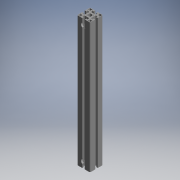
# Autodesk Inventor part: HFS8-5050-500-LSV-RSV
Saved by Autodesk Inventor 2017.3 (Build 213256000, 256)
## iProperties
Part Number: HFS8-5050-500-LSV-RSV
Material: Generic
Catalog Web Link: www.cadenas.de
Description: NEFS8-5050, EFS8-5050, EFSB8-5050, HFS8-5050, HFSB8-5050, GFS8-5050, HFSF8-5050, HFST8-5050-HFS8 Series Aluminum Extrusions 50 Square -1 Slot-
Vendor: MISUMI
Document SubType Name: Modeling
Designer: partserver
Manufacturer: MISUMI
Mass: 622.053 g
Surface Area: 2899.68 cm^2
Volume: 622.053 cm^3
Density: 1 g/cm^3
Appearance: PSOLRGB-175-175-175
Category: PARTsolutions
Company: MISUMI
Title: HFS8-5050-500-LSV-RSV
Author: Cadenas PARTsolutions
Comments: HFS8 Series Aluminum Extrusions 50 Square -1 Slot-
PSOL_IDENT_0: {$CADENAS_DATA\23d-libs\misumi\metric\38_al_extrusions_blackets\8_45\hfs8_5050.prj},643 {VTYP=3D},{N
PSOL_IDENT_1: B=HFS8-5050-500-LSV-RSV},{LINA=HFS8-5050-500-LSV-RSV},{NN=NEFS8-5050, EFS8-5050, EFSB8-5050, HFS8-50
PSOL_IDENT_2: 50, HFSB8-5050, GFS8-5050, HFSF8-5050, HFST8-5050},{DATE=08.06.2021 08:26:18},{GEOMDATE=13.07.2020 0
PSOL_IDENT_3: 4:45:18},{VERSION=},{LINEID=130},{WBVAR=L,ALT1,ALT2,ALT4,ALT5,CP5,DL5,DR5,ALT6,ALT9,ALT10,ALT11,HP6,
PSOL_IDENT_4: NHL6,DL6,NHR6,DR6,ALT7,ALT8,NH9,AH,BH,CH,DH,EH,NH10,AV,BV,CV,DV,EV,NH11,AP,BP,CP,DP,EP,ALT12,ALT13,Z
PSOL_IDENT_5: ,NH12,XA,XB,XC,XD,XE,NH13,YA,YB,YC,YD,YE,ALT14,HP14,DL14,DR14,ALT15,HP15,DL15,DR15,ALT16,HP16,DL16,D
PSOL_IDENT_6: R16,ALT19,ALT20},{WBNUMERIC=L,NH9,AH,BH,CH,DH,EH,NH10,AV,BV,CV,DV,EV,NH11,AP,BP,CP,DP,EP,NH12,XA,XB,
PSOL_IDENT_7: XC,XD,XE,NH13,YA,YB,YC,YD,YE}  {NB=HFS8-5050-500-LSV-RSV},{LINA=HFS8-5050-500-LSV-RSV},{KT=DUMMY},{P
PSOL_IDENT_8: N=HFS8-5050-500-LSV-RSV},{TPS=HFS8-5050},{MAT=A6N01SS-T5 Aluminum Alloy},{ST=Clear Anodize},{FRMW=50
PSOL_IDENT_9: },{FRMH=50},{FRD=12.5},{L=500.0},{MASS=3.43},{SA=1150},{LX=26.64x10^4},{LY=26.64x10^4},{ALT1=},{M1=0
PSOL_IDENT_10: },{IDM1=10.106},{DPL1=0},{DPR1=0},{ALT1PN=},{ALT2=},{ALT2ALG= '','w/o End Tapping (Heli-Coil Insert)'
PSOL_IDENT_11: ,'LHP','with LHP (Tapping on the Left (Heli-Coil Insert))','RHP','with RHP (Tapping on the Right (He
PSOL_IDENT_12: li-Coil Insert))','HPW','with HPW (Tapping on Both Ends (Heli-Coil Insert))' },{M2=0},{DP2=0},{ALT2P
PSOL_IDENT_13: N=},{ALT4=},{ALT4ALG= '', 'w/o SC (High Precision Cut)', 'SC', 'with SC (High Precision Cut)' },{ALT
PSOL_IDENT_14: 4PN=},{ALT5=},{ALT5ALG= '','w/o 45 Degree Cut','1','with 45 Degree Cut' },{CP5=},{CP5ALG= '','N/A' }
PSOL_IDENT_15: ,{DL5=},{DL5ALG= '','N/A' },{DR5=},{DR5ALG= '','N/A' },{FRMLALT5=0},{FRMRALT5=0},{ALT5PN=},{ALT6=},{
PSOL_IDENT_16: ALT6ALG= '','w/o Fastening Location Wrench Access Hole Alterations','1','with Fastening Location Wre
PSOL_IDENT_17: nch Access Hole Alterations' },{ALT9=},{ALT9ALG= '','w/o Location Specified Wrench Access Hole Alter
PSOL_IDENT_18: atons (Horizontal)','1','with Location Specified Wrench Access Hole Alteratons (Horizontal)' },{ALT1
PSOL_IDENT_19: 0=},{ALT10ALG= '','w/o Location Specified Wrench Access Hole Alteratons (Vertical)','1','with Locati
PSOL_IDENT_20: on Specified Wrench Access Hole Alteratons (Vertical)' },{ALT11=},{ALT11ALG= '','w/o Location Specif
PSOL_IDENT_21: ied Wrench Access Hole Alteratons (Crisscross)','1','with Location Specified Wrench Access Hole Alte
PSOL_IDENT_22: ratons (Crisscross)' },{HP6=},{HP6ALG= '','N/A' },{NHL6=},{NHL6ALG= '','N/A' },{DL6=},{DL6ALG= '','N
PSOL_IDENT_23: /A' },{NHR6=},{NHR6ALG= '','N/A' },{DR6=},{DR6ALG= '','N/A' },{HL6=0.0},{HL6D=0.0},{HR6=0.0},{HR6D=0
PSOL_IDENT_24: .0},{J6=0},{J6D=0},{K6=0},{K6D=0},{DD6=0},{DD6ALG=0},{ALT7=},{ALT7ALG= '','N/A' },{ALT8=},{ALT8ALG= ''
PSOL_IDENT_25: ,'N/A' },{ALT678PN=},{NH9=0},{NH9MAX=5},{NH9ALG=[0]},{AH=0.0},{AHMIN=7},{AHMAX=495},{AHALG=[0]},{BH=
PSOL_IDENT_26: 0.0},{BHMIN=2},{BHMAX=497},{BHALG=[0]},{CH=0.0},{CHMIN=2},{CHMAX=499},{CHALG=[0]},{DH=0.0},{DHMIN=2}
PSOL_IDENT_27: ,{DHMAX=501},{DHALG=[0]},{EH=0.0},{EHMIN=2},{EHMAX=493},{EHALG=[0]},{NH10=0},{NH10MAX=5},{NH10ALG=[0
PSOL_IDENT_28: ]},{AV=0.0},{AVMIN=7},{AVMAX=495},{AVALG=[0]},{BV=0.0},{BVMIN=2},{BVMAX=497},{BVALG=[0]},{CV=0.0},{C
PSOL_IDENT_29: VMIN=2},{CVMAX=499},{CVALG=[0]},{DV=0.0},{DVMIN=2},{DVMAX=501},{DVALG=[0]},{EV=0.0},{EVMIN=2},{EVMAX=
PSOL_IDENT_30: 493},{EVALG=[0]},{NH11=0},{NH11MAX=5},{NH11ALG=[0]},{AP=0.0},{APMIN=7},{APMAX=495},{APALG=[0]},{BP=0
PSOL_IDENT_31: .0},{BPMIN=2},{BPMAX=497},{BPALG=[0]},{CP=0.0},{CPMIN=2},{CPMAX=499},{CPALG=[0]},{DP=0.0},{DPMIN=2},
PSOL_IDENT_32: {DPMAX=501},{DPALG=[0]},{EP=0.0},{EPMIN=2},{EPMAX=493},{EPALG=[0]},{ALT9PN=},{ALT10PN=},{ALT11PN=},{
PSOL_IDENT_33: ALT91011PN=},{ALT12=},{ALT12ALG= '','w/o Counterbore Hole in Specified Position (Vertical)','1','wit
PSOL_IDENT_34: h Counterbore Hole in Specified Position (Vertical)' },{ALT13=},{ALT13ALG= '','w/o Counterbore Hole
PSOL_IDENT_35: in Specified Position (Horizontal)','1','with Counterbore Hole in Specified Position (Horizontal)' }
PSOL_IDENT_36: ,{Z=},{ZALG= '','N/A' },{DD12=0.0},{DD112=0},{NH12=0},{NH12MAX=5},{NH12ALG=[0]},{XA=0.0},{XAMIN=7},{
PSOL_IDENT_37: XAMAX=495},{XAALG=[0]},{XB=0.0},{XBMIN=2},{XBMAX=497},{XBALG=[0]},{XC=0.0},{XCMIN=2},{XCMAX=499},{XC
PSOL_IDENT_38: ALG=[0]},{XD=0.0},{XDMIN=2},{XDMAX=501},{XDALG=[0]},{XE=0.0},{XEMIN=2},{XEMAX=493},{XEALG=[0]},{NH13=
PSOL_IDENT_39: 0},{NH13MAX=5},{NH13ALG=[0]},{YA=0.0},{YAMIN=7},{YAMAX=495},{YAALG=[0]},{YB=0.0},{YBMIN=2},{YBMAX=49
PSOL_IDENT_40: 7},{YBALG=[0]},{YC=0.0},{YCMIN=2},{YCMAX=499},{YCALG=[0]},{YD=0.0},{YDMIN=2},{YDMAX=501},{YDALG=[0]}
PSOL_IDENT_41: ,{YE=0.0},{YEMIN=2},{YEMAX=493},{YEALG=[0]},{ALT12PN=},{ALT13PN=},{ALT1213PN=},{ALT14=},{ALT14ALG= ''
PSOL_IDENT_42: ,'w/o D Type Hole Alteration','1','with D Type Hole Alteration' },{HP14=},{HP14ALG= '','N/A' },{DL14=
PSOL_IDENT_43: },{DL14ALG= '','N/A' },{DR14=},{DR14ALG= '','N/A' },{H14=0.0},{D14=0.0},{ALT14PN=},{ALT15=1},{ALT15A
PSOL_IDENT_44: LG= '','w/o S Type Hole Alteration','1','with S Type Hole Alteration' },{HP15=LR},{HP15ALG= 'L','Lef
PSOL_IDENT_45: t','R','Right','LR','Both Sides' },{DL15=V},{DL15ALG= 'H','Horizontal','V','Vertical','P','Crisscros
PSOL_IDENT_46: s' },{DR15=V},{DR15ALG= 'H','Horizontal','V','Vertical','P','Crisscross' },{H15=22.5},{D115=20},{D21
PSOL_IDENT_47: 5=15.1},{ALT15PN=-LSV-RSV},{ALT16=},{ALT16ALG= '','w/o M Type Hole Alteration','1','with M Type Hole
PSOL_IDENT_48: Alteration' },{HP16=},{HP16ALG= '','N/A' },{DL16=},{DL16ALG= '','N/A' },{DR16=},{DR16ALG= '','N/A'
PSOL_IDENT_49: },{H116=0},{D16=0.0},{ALT16PN=},{ALT19=},{ALT19ALG= '','N/A' },{M19=0},{DP19=0},{ALT19PN=},{ALT20=},
PSOL_IDENT_50: {ALT20PN=},{ERRORALT01=OK},{ERRORALT02=OK},{ERRORALT05=OK},{ERRORALT06091=OK},{ERRORALT06092=OK},{ER
PSOL_IDENT_51: RORALT06093=OK},{ERRORALT06094=OK},{ERRORALT06101=OK},{ERRORALT06102=OK},{ERRORALT06103=OK},{ERRORAL
PSOL_IDENT_52: T06104=OK},{ERRORALT06111=OK},{ERRORALT06112=OK},{ERRORALT06113=OK},{ERRORALT06114=OK},{ERRORALT0612
PSOL_IDENT_53: 1=OK},{ERRORALT06122=OK},{ERRORALT06123=OK},{ERRORALT06124=OK},{ERRORALT06131=OK},{ERRORALT06132=OK}
PSOL_IDENT_54: ,{ERRORALT06133=OK},{ERRORALT06134=OK},{ERRORALT0614=OK},{ERRORALT0615=OK},{ERRORALT0616=OK},{ERRORA
PSOL_IDENT_55: LT0619=OK},{ERRORALT0911=OK},{ERRORALT0913=OK},{ERRORALT0914=OK},{ERRORALT0915=OK},{ERRORALT0916=OK}
PSOL_IDENT_56: ,{ERRORALT0919=OK},{ERRORALT1011=OK},{ERRORALT1012=OK},{ERRORALT1014=OK},{ERRORALT1015=OK},{ERRORALT
PSOL_IDENT_57: 1016=OK},{ERRORALT1019=OK},{ERRORALT1112=OK},{ERRORALT1113=OK},{ERRORALT1114=OK},{ERRORALT1115=OK},{
PSOL_IDENT_58: ERRORALT1116=OK},{ERRORALT1119=OK},{ERRORALT1214=OK},{ERRORALT1215=OK},{ERRORALT1216=OK},{ERRORALT12
PSOL_IDENT_59: 19=OK},{ERRORALT1314=OK},{ERRORALT1315=OK},{ERRORALT1316=OK},{ERRORALT1319=OK},{ERRORALT1415=OK},{ER
PSOL_IDENT_60: RORALT1416=OK},{ERRORALT1419=OK},{ERRORALT1516=OK},{ERRORALT1519=OK},{ERRORALT1619=OK},{ERRORPN=},{T
PSOL_IDENT_61: FH=0},{TFW=0}
NB: HFS8-5050-500-LSV-RSV
NN: NEFS8-5050, EFS8-5050, EFSB8-5050, HFS8-5050, HFSB8-5050, GFS8-5050, HFSF8-5050, HFST8-5050
NT: HFS8 Series Aluminum Extrusions 50 Square -1 Slot-
NBSYN: $PN.
LINA: HFS8-5050-500-LSV-RSV
CATALOG: Misumi
PN: HFS8-5050-500-LSV-RSV
TPS: HFS8-5050
MAT: A6N01SS-T5 Aluminum Alloy
ST: Clear Anodize
L: 500
MASS: 3.43
SA: 1150
LX: 26.64x10^4
LY: 26.64x10^4
ALT1: w/o End Tapping
M1: 0
DPL1: 0
DPR1: 0
ALT2: w/o End Tapping (Heli-Coil Insert)
M2: 0
DP2: 0
ALT4: w/o SC (High Precision Cut)
ALT5: w/o 45 Degree Cut
CP5: N/A
DL5: N/A
DR5: N/A
ALT6: w/o Fastening Location Wrench Access Hole Alterations
ALT9: w/o Location Specified Wrench Access Hole Alteratons (Horizontal)
ALT10: w/o Location Specified Wrench Access Hole Alteratons (Vertical)
ALT11: w/o Location Specified Wrench Access Hole Alteratons (Crisscross)
HP6: N/A
NHL6: N/A
DL6: N/A
NHR6: N/A
DR6: N/A
HL6D: 0
HR6D: 0
J6D: 0
K6D: 0
DD6: 0
ALT7: N/A
ALT8: N/A
NH9: 0
AH: 0
BH: 0
CH: 0
DH: 0
EH: 0
NH10: 0
AV: 0
BV: 0
CV: 0
DV: 0
EV: 0
NH11: 0
AP: 0
BP: 0
CP: 0
DP: 0
EP: 0
ALT12: w/o Counterbore Hole in Specified Position (Vertical)
ALT13: w/o Counterbore Hole in Specified Position (Horizontal)
Z: N/A
DD12: 0
DD112: 0
NH12: 0
XA: 0
XB: 0
XC: 0
XD: 0
XE: 0
NH13: 0
YA: 0
YB: 0
YC: 0
YD: 0
YE: 0
ALT14: w/o D Type Hole Alteration
HP14: N/A
DL14: N/A
DR14: N/A
H14: 0
D14: 0
ALT15: with S Type Hole Alteration
HP15: Both Sides
DL15: Vertical
DR15: Vertical
H15: 22.5
D115: 20
D215: 15.1
ALT16: w/o M Type Hole Alteration
HP16: N/A
DL16: N/A
DR16: N/A
H116: 0
D16: 0
ALT19: N/A
M19: 0
DP19: 0
ALT20: w/o CW (End Face C Chamfering)
SUPPLIER: MISUMI
ARTICLENO: HFS8-5050-500-LSV-RSV
BOMINFO: HFS8-5050-500-LSV-RSV
CREATOR: CADENAS GmbH
Autodesk Inventor part; units mm, degrees
ref_plane "YZ Plane" through (0, 0, 0) normal (1, 0, 0) x (0, 1, 0)
ref_plane "XZ Plane" through (0, 0, 0) normal (0, 1, 0) x (-1, 0, 0)
ref_plane "XY Plane" through (0, 0, 0) normal (0, 0, 1) x (1, 0, 0)
sketch "Sketch_1" plane through (0, 0, 0) normal (0, 0, 1) x (1, 0, 0)
  line L0 (-25, -5) -> (-25, -22)
  arc A0 (-25, -22) -> (-22, -25) centre (-22, -22) ccw
  line L1 (-22, -25) -> (-5, -25)
  line L2 (-5, -25) -> (-5, -19)
  line L3 (-5, -19) -> (-10, -19)
  line L4 (-10, -19) -> (-10, -14.5962)
  line L5 (-10, -14.5962) -> (-7.4038, -12)
  line L6 (-7.4038, -12) -> (-1.2124, -12)
  line L7 (-1.2124, -12) -> (0, -11.3)
  line L8 (0, -11.3) -> (1.2124, -12)
  line L9 (1.2124, -12) -> (7.4038, -12)
  line L10 (7.4038, -12) -> (10, -14.5962)
  line L11 (10, -14.5962) -> (10, -19)
  line L12 (10, -19) -> (5, -19)
  line L13 (5, -19) -> (5, -25)
  line L14 (5, -25) -> (22, -25)
  arc A1 (22, -25) -> (25, -22) centre (22, -22) ccw
  line L15 (25, -22) -> (25, -5)
  line L16 (25, -5) -> (19, -5)
  line L17 (19, -5) -> (19, -10)
  line L18 (19, -10) -> (14.5962, -10)
  line L19 (14.5962, -10) -> (12, -7.4038)
  line L20 (12, -7.4038) -> (12, -1.2124)
  line L21 (12, -1.2124) -> (11.3, 0)
  line L22 (11.3, 0) -> (12, 1.2124)
  line L23 (12, 1.2124) -> (12, 7.4038)
  line L24 (12, 7.4038) -> (14.5962, 10)
  line L25 (14.5962, 10) -> (19, 10)
  line L26 (19, 10) -> (19, 5)
  line L27 (19, 5) -> (25, 5)
  line L28 (25, 5) -> (25, 22)
  arc A2 (25, 22) -> (22, 25) centre (22, 22) ccw
  line L29 (22, 25) -> (5, 25)
  line L30 (5, 25) -> (5, 19)
  line L31 (5, 19) -> (10, 19)
  line L32 (10, 19) -> (10, 14.5962)
  line L33 (10, 14.5962) -> (7.4038, 12)
  line L34 (7.4038, 12) -> (1.2124, 12)
  line L35 (1.2124, 12) -> (0, 11.3)
  line L36 (0, 11.3) -> (-1.2124, 12)
  line L37 (-1.2124, 12) -> (-7.4038, 12)
  line L38 (-7.4038, 12) -> (-10, 14.5962)
  line L39 (-10, 14.5962) -> (-10, 19)
  line L40 (-10, 19) -> (-5, 19)
  line L41 (-5, 19) -> (-5, 25)
  line L42 (-5, 25) -> (-22, 25)
  arc A3 (-22, 25) -> (-25, 22) centre (-22, 22) ccw
  line L43 (-25, 22) -> (-25, 5)
  line L44 (-25, 5) -> (-19, 5)
  line L45 (-19, 5) -> (-19, 10)
  line L46 (-19, 10) -> (-14.5962, 10)
  line L47 (-14.5962, 10) -> (-12, 7.4038)
  line L48 (-12, 7.4038) -> (-12, 1.2124)
  line L49 (-12, 1.2124) -> (-11.3, 0)
  line L50 (-11.3, 0) -> (-12, -1.2124)
  line L51 (-12, -1.2124) -> (-12, -7.4038)
  line L52 (-12, -7.4038) -> (-14.5962, -10)
  line L53 (-14.5962, -10) -> (-19, -10)
  line L54 (-19, -10) -> (-19, -5)
  line L55 (-19, -5) -> (-25, -5)
  arc A4 (14.5, 23) -> (14.5, 21) centre (14.5, 22) ccw
  line L56 (14.5, 21) -> (14.5, 15.5)
  arc A5 (14.5, 15.5) -> (15.5, 14.5) centre (15.5, 15.5) ccw
  line L57 (15.5, 14.5) -> (21, 14.5)
  arc A6 (21, 14.5) -> (23, 14.5) centre (22, 14.5) ccw
  line L58 (23, 14.5) -> (23, 22)
  arc A7 (23, 22) -> (22, 23) centre (22, 22) ccw
  line L59 (22, 23) -> (14.5, 23)
  arc A8 (14.5, -21) -> (14.5, -23) centre (14.5, -22) ccw
  line L60 (14.5, -23) -> (22, -23)
  arc A9 (22, -23) -> (23, -22) centre (22, -22) ccw
  line L61 (23, -22) -> (23, -14.5)
  arc A10 (23, -14.5) -> (21, -14.5) centre (22, -14.5) ccw
  line L62 (21, -14.5) -> (15.5, -14.5)
  arc A11 (15.5, -14.5) -> (14.5, -15.5) centre (15.5, -15.5) ccw
  line L63 (14.5, -15.5) -> (14.5, -21)
  line L64 (-23, 22) -> (-23, 14.5)
  arc A12 (-23, 14.5) -> (-21, 14.5) centre (-22, 14.5) ccw
  line L65 (-21, 14.5) -> (-15.5, 14.5)
  arc A13 (-15.5, 14.5) -> (-14.5, 15.5) centre (-15.5, 15.5) ccw
  line L66 (-14.5, 15.5) -> (-14.5, 21)
  arc A14 (-14.5, 21) -> (-14.5, 23) centre (-14.5, 22) ccw
  line L67 (-14.5, 23) -> (-22, 23)
  arc A15 (-22, 23) -> (-23, 22) centre (-22, 22) ccw
  line L68 (-23, -14.5) -> (-23, -22)
  arc A16 (-23, -22) -> (-22, -23) centre (-22, -22) ccw
  line L69 (-22, -23) -> (-14.5, -23)
  arc A17 (-14.5, -23) -> (-14.5, -21) centre (-14.5, -22) ccw
  line L70 (-14.5, -21) -> (-14.5, -15.5)
  arc A18 (-14.5, -15.5) -> (-15.5, -14.5) centre (-15.5, -15.5) ccw
  line L71 (-15.5, -14.5) -> (-21, -14.5)
  arc A19 (-21, -14.5) -> (-23, -14.5) centre (-22, -14.5) ccw
  constraints: 144 end point, 40 point on circle, 20 centre point
extrude "Extrusion1" add sketch "Sketch_1" against normal blind 500
sketch "Sketch_87" plane through (0, 0, 0) normal (0, 0, 1) x (1, 0, 0)
  arc A0 (-5.9646, -4.5504) -> (-4.5504, -5.9646) centre (-6, -6) ccw
  line L0 (-4.5504, -5.9646) -> (-3.9465, -5.3607)
  arc A1 (-3.3268, -5.291) -> (-3.9465, -5.3607) centre (-3.593, -5.7143) ccw
  arc A2 (-3.3268, -5.291) -> (3.3268, -5.291) centre (0, 0) ccw
  arc A3 (3.9465, -5.3607) -> (3.3268, -5.291) centre (3.593, -5.7143) ccw
  line L1 (3.9465, -5.3607) -> (4.5504, -5.9646)
  arc A4 (4.5504, -5.9646) -> (5.9646, -4.5504) centre (6, -6) ccw
  line L2 (5.9646, -4.5504) -> (5.3607, -3.9465)
  arc A5 (5.291, -3.3268) -> (5.3607, -3.9465) centre (5.7143, -3.593) ccw
  arc A6 (5.291, -3.3268) -> (5.291, 3.3268) centre (0, 0) ccw
  arc A7 (5.3607, 3.9465) -> (5.291, 3.3268) centre (5.7143, 3.593) ccw
  line L3 (5.3607, 3.9465) -> (5.9646, 4.5504)
  arc A8 (5.9646, 4.5504) -> (4.5504, 5.9646) centre (6, 6) ccw
  line L4 (4.5504, 5.9646) -> (3.9465, 5.3607)
  arc A9 (3.3268, 5.291) -> (3.9465, 5.3607) centre (3.593, 5.7143) ccw
  arc A10 (3.3268, 5.291) -> (-3.3268, 5.291) centre (0, 0) ccw
  arc A11 (-3.9465, 5.3607) -> (-3.3268, 5.291) centre (-3.593, 5.7143) ccw
  line L5 (-3.9465, 5.3607) -> (-4.5504, 5.9646)
  arc A12 (-4.5504, 5.9646) -> (-5.9646, 4.5504) centre (-6, 6) ccw
  line L6 (-5.9646, 4.5504) -> (-5.3607, 3.9465)
  arc A13 (-5.291, 3.3268) -> (-5.3607, 3.9465) centre (-5.7143, 3.593) ccw
  arc A14 (-5.291, 3.3268) -> (-5.291, -3.3268) centre (0, 0) ccw
  arc A15 (-5.3607, -3.9465) -> (-5.291, -3.3268) centre (-5.7143, -3.593) ccw
  line L7 (-5.3607, -3.9465) -> (-5.9646, -4.5504)
  constraints: 32 point on circle, 16 centre point, 16 end point
extrude "Extrusion2" cut sketch "Sketch_87" against normal blind 500
sketch "Sketch_71" plane through (0, 0, 0) normal (1, 0, 0) x (0, 0, -1)
  line L0 (22.5, -25) -> (22.5, 25)
  line L1 (22.5, 25) -> (32.5, 25)
  line L2 (32.5, 25) -> (32.5, 19)
  line L3 (32.5, 19) -> (30.05, 19)
  line L4 (30.05, 19) -> (30.05, -19)
  line L5 (30.05, -19) -> (32.5, -19)
  line L6 (32.5, -19) -> (32.5, -25)
  line L7 (32.5, -25) -> (22.5, -25)
  line L8 (22.5, -25) -> (22.5, 25)
  constraints: 18 end point
revolve "Revolution1" cut sketch "Sketch_71" angle 360 about axis through (0, -25, -22.5) along (0, -1, 0)
sketch "Sketch_72" plane through (0, 0, 0) normal (1, 0, 0) x (0, 0, -1)
  line L0 (477.5, -25) -> (477.5, 25)
  line L1 (477.5, 25) -> (487.5, 25)
  line L2 (487.5, 25) -> (487.5, 19)
  line L3 (487.5, 19) -> (485.05, 19)
  line L4 (485.05, 19) -> (485.05, -19)
  line L5 (485.05, -19) -> (487.5, -19)
  line L6 (487.5, -19) -> (487.5, -25)
  line L7 (487.5, -25) -> (477.5, -25)
  line L8 (477.5, -25) -> (477.5, 25)
  constraints: 18 end point
revolve "Revolution2" cut sketch "Sketch_72" angle 360 about axis through (0, -25, -477.5) along (0, -1, 0)
ref_plane "C1_XY" through (0, 0, 0) normal (0, 0, 1) x (1, 0, 0)
ref_plane "C1_YZ" through (0, 0, 0) normal (1, 0, 0) x (0, 1, 0)
ref_plane "C1_ZX" through (0, 0, 0) normal (0, 1, 0) x (0, 0, 1)
ref_plane "to_frame_cap1_XY" through (0, 0, 0) normal (0, 0, 1) x (1, 0, 0)
ref_plane "to_frame_cap1_YZ" through (0, 0, 0) normal (1, 0, 0) x (0, 1, 0)
ref_plane "to_frame_cap1_ZX" through (0, 0, 0) normal (0, 1, 0) x (0, 0, 1)
ref_plane "to_frame_cap2_XY" through (0, 0, -500) normal (0, 0, -1) x (1, 0, 0)
ref_plane "to_frame_cap2_YZ" through (0, 0, -500) normal (1, 0, 0) x (0, -1, 0)
ref_plane "to_frame_cap2_ZX" through (0, 0, -500) normal (0, -1, 0) x (0, 0, -1)
body "Solid1"
